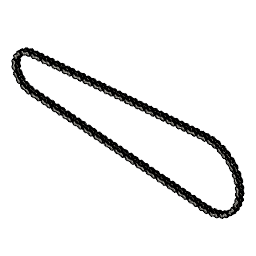
2410994757_Bicycle-Chain (Autodesk Fusion 360 design; units mm, degrees)
part number: 2025-11-01-18-05-41-506
Autodesk Fusion 360 part; units mm, degrees
note: some values were not read from the file. Chosen so that the rebuilt part matches the saved one: a direction; which bodies a step acts on. Set by a fixed rule: which sketch regions a step uses.
sketch "Sketch4" plane through (0, 0, 0) normal (0, 1, 0) x (1, 0, 0)
  line L0 (0, 0) -> (0, -57.0944)
  line L1 (0, 0) -> (-8.7438, -55.2063)
  line L2 (0, 0) -> (8.7438, -55.2063)
  circle A0 centre (0, 0) radius 37.5
  circle A1 centre (-5.8663, -37.0383) radius 4.5
  circle A2 centre (5.8663, -37.0383) radius 4.5
  line L3 (-5.8663, -37.0383) -> (5.8663, -37.0383)
  circle A3 centre (0, -44.8261) radius 5.25
  circle A4 centre (0, -29.2506) radius 5.25
  circle A5 centre (-5.8663, -37.0383) radius 3
  circle A6 centre (-5.8663, -37.0383) radius 2.25
  circle A7 centre (5.8663, -37.0383) radius 2.25
  circle A8 centre (5.8663, -37.0383) radius 3
  dimension "d26" = 9
  dimension "d27" = 9
  dimension "d28" = 75
  dimension "d29" = 9
  dimension "d30" = 10.5
  dimension "d31" = 6
  dimension "d32" = 4.5
  constraint coincident L0.start L1.start
  constraint vertical L0
  constraint coincident A0 A1.centre
  constraint coincident L1 A1.centre
  constraint symmetric L0 A1 A2
  constraint coincident A1.centre L3.start
  constraint coincident A2.centre L3.end
  constraint coincident L0 A3.centre
  constraint tangent A1 A3
  constraint symmetric L3 A3 A4
  constraint concentric A1 A5
  constraint concentric A5 A6
  constraint symmetric L0 A5 A8
  constraint symmetric L0 A6 A7
  measures "d26" angle of L0 L1
  measures "d27" angle of L0 L2
  measures "d28" diameter of A0
  measures "d29" diameter of A1
  measures "d30" diameter of A3
  measures "d31" diameter of A5
  measures "d32" diameter of A6
extrude "Extrude5" add sketch "Sketch4" along normal blind 1.5 contours L0 A2 L3 A4 | L0 A1 L3 A4 | L0 A0 A2 L3 | L0 A0 A1 L3 | L1 A1 L3 A5 | L2 A2 L3 A8 | L1 A0 A1 A5 | L2 A0 A2 A8 | L0 A0 A2 A3 | L0 A0 A1 A3 | A0 A1 L3 A5 | A0 A2 L3 A8 | L1 L3 A5 A6 | L1 A0 A5 A6 | L1 A0 A1 A5 | L2 A0 A7 A8 | L2 L3 A7 A8 | L2 A0 A2 A8 | L1 A0 A1 A5 | L2 A0 A2 A8 | A0 L3 A5 A6 | A0 L3 A7 A8 | L1 A0 A5 A6 | L2 A0 A7 A8 | L1 A0 A5 A6 | L2 A0 A7 A8 makes body 1
extrude "Extrude6" add sketch "Sketch4" along normal mid plane 10.5 separate body contours L1 L3 A6 | L1 A0 A6 | L2 A0 A7 | L2 L3 A7 | A0 L3 A6 | A0 L3 A7 | L1 A0 A6 | L1 A0 A6 | L2 A0 A7 | L2 A0 A7 makes body 2 at (-3.6275, 1.75, 36.8143) makes body 3 at (3.6191, 1.75, 36.9262)
move_body "Align1" bodies 1 to x (1, 0, 0) y (0, 1, 0) z (0, 0, 1) at (0, 3.75, 0)
mirror "Mirror1" about plane through (0, 0, 0) normal (0, 1, 0) of bodies 1 makes body 4
extrude "Extrude7" add sketch "Sketch4" along normal blind 1.5 separate body contours L0 A2 L3 A4 | L0 A1 L3 A4 | L0 A0 A2 L3 | L0 A0 A1 L3 | L1 A1 L3 A5 | L2 A2 L3 A8 | L1 A0 A1 A5 | L2 A0 A2 A8 | L0 A0 A2 A3 | L0 A0 A1 A3 | A0 A1 L3 A5 | A0 A2 L3 A8 | L1 A0 A1 A5 | L2 A0 A2 A8 | L1 A0 A1 A5 | L2 A0 A2 A8 makes body 5
extrude "Extrude8" add sketch "Sketch4" along normal mid plane 7.5 separate body contours L1 L3 A5 A6 | L1 A0 A5 A6 | L2 A0 A7 A8 | L2 L3 A7 A8 | A0 L3 A5 A6 | A0 L3 A7 A8 | L1 A0 A5 A6 | L2 A0 A7 A8 | L1 A0 A5 A6 | L2 A0 A7 A8 makes body 6 at (-2.9075, 2.5, 37.5337) makes body 7 at (8.8514, -1.25, 37.337)
move_body "Align2" bodies 5 to x (1, 0, 0) y (0, 1, 0) z (0, 0, 1) at (0, 2.25, 0)
mirror "Mirror2" about plane through (0, 0, 0) normal (0, 1, 0) of bodies 5 makes body 8
combine "Combine2" operation add target body 5 tool bodies 6 7 8
combine "Combine3" operation add target body 1 tool bodies 2 3 4
move_body "Move1" bodies 1 to x (0.951057, 0, -0.309017) y (0, 1, 0) z (0.309017, 0, 0.951057) at (0, 0, 0)
pattern_circular "C-Pattern2" count 6 over 180 about axis through (0, 0, 0) along (0, -1, 0) of bodies 1 5 makes body 9 at (-17.1688, -5.25, 33.5877) makes body 10 at (-33.5487, -5.25, 17.5808) makes body 11 at (-37.1681, 5.25, 6.1192) makes body 12 at (-27.0874, -5.25, -26.4739) makes body 13 at (-16.7873, -5.25, -33.7221) makes body 14 at (-22.5435, -2.25, 29.403) makes body 15 at (-34.8528, 2.25, 12.5927) makes body 16 at (-34.9303, -2.25, -12.3541) makes body 17 at (-20.9976, -2.25, -30.5262) makes body 18 at (-1.2063, 2.25, -37.0383)
sketch "Sketch5" plane through (0, 0, 0) normal (0, 1, 0) x (1, 0, 0)
  line L0 (0, 0) -> (400, 0)
  line L1 (-3.0469, -37.376) -> (394.3125, -69.7686)
  line L2 (-3.0469, 37.376) -> (394.3125, 69.7686)
  arc A0 (-3.0469, 37.376) -> (-3.0469, -37.376) centre (0, 0) ccw
  arc A1 (394.3125, -69.7686) -> (394.3125, 69.7686) centre (400, 0) ccw
  dimension "d68" = 75
  dimension "d69" = 400
  dimension "d70" = 140
  constraint coincident L0.start A0.centre
  constraint horizontal L0
  constraint coincident L0.end A1.centre
  constraint tangent L1 A0
  constraint tangent L1 A1
  constraint tangent L2 A1
  constraint tangent L2 A0
  measures "d68" diameter of A0
  measures "d69" distance of L0.start L0.end
  measures "d70" diameter of A1
move_body "Move2" bodies 1 to x (1, 0, 0) y (0, 1, 0) z (0, 0, 1) at (100, 0, 0)
move_body "Move3" bodies 5 to x (0.996195, 0, 0.087156) y (0, 1, 0) z (-0.087156, 0, 0.996195) at (2.7965, 0, 1.0273)
move_body "Move4" bodies 5 to x (1, 0, 0) y (0, 1, 0) z (0, 0, 1) at (0.4623, 0, -0.4202)
move_body "Move5" bodies 5 to x (0.999848, 0, 0.017452) y (0, 1, 0) z (-0.017452, 0, 0.999848) at (0.6455, 0, 0.108)
move_body "Move6" bodies 1 to x (1, 0, 0) y (0, 1, 0) z (0, 0, 1) at (-100.03, 0, 1.1325)
move_body "Move7" bodies 1 to x (0.913545, 0, 0.406737) y (0, 1, 0) z (-0.406737, 0, 0.913545) at (16.03, 0, 0.9262)
copy_body "CopyPasteBodies1" bodies 5 makes body 19
move_body "Move8" bodies 19 to x (1, 0, 0) y (0, 1, 0) z (0, 0, 1) at (23.3209, 0, 2.4356)
move_body "Move9" bodies 19 to x (0.999848, 0, -0.017452) y (0, 1, 0) z (0.017452, 0, 0.999848) at (-0.6855, 0, 0.3116)
move_body "Move26" bodies 19 to x (0.999848, 0, -0.017452) y (0, 1, 0) z (0.017452, 0, 0.999848) at (-0.6855, 0, 0.3116)
pattern_path "PathPattern3" count 16 spacing 23.5684 from (17.537, 0, 39.054) backwards path "Sketch5" along L2 A0 L1 A1 of bodies 1 19 makes body 20 at (29.7958, 5.25, 40.9755) makes body 21 at (52.9479, 5.25, 41.8939) makes body 22 at (76.8225, 5.25, 43.3228) makes body 23 at (100.0948, 5.25, 46.0838) makes body 24 at (134.64, 5.25, 49.465) makes body 25 at (146.8849, 5.25, 49.792) makes body 26 at (170.3753, 5.25, 51.7069) makes body 27 at (193.6488, 5.25, 53.9127) makes body 28 at (217.1393, 5.25, 55.8276) makes body 29 at (240.6297, 5.25, 57.7425) makes body 30 at (275.398, -5.25, 59.2453) makes body 31 at (298.8885, -5.25, 61.1603) makes body 32 at (324.347, 5.25, 65.2814) makes body 33 at (345.9825, 5.25, 65.0292) makes body 34 at (370.9655, 5.25, 70.5162) makes body 35 at (48.3035, 3.75, 41.8554) makes body 36 at (71.794, 3.75, 43.7704) makes body 37 at (95.2845, 3.75, 45.6853) makes body 38 at (118.775, 3.75, 47.6002) makes body 39 at (142.2655, 3.75, 49.5152) makes body 40 at (165.756, 3.75, 51.4301) makes body 41 at (189.2465, 3.75, 53.345) makes body 42 at (212.737, 3.75, 55.26) makes body 43 at (236.2275, 3.75, 57.1749) makes body 44 at (259.718, 3.75, 59.0898) makes body 45 at (283.2085, 3.75, 61.0048) makes body 46 at (306.6989, 3.75, 62.9197) makes body 47 at (330.1894, 3.75, 64.8346) makes body 48 at (353.6799, 3.75, 66.7496) makes body 49 at (377.1704, 3.75, 68.6645)
copy_body "CopyPasteBodies8" bodies 49 makes body 50
move_body "Move27" bodies 50 to x (1, 0, 0) y (0, 1, 0) z (0, 0, 1) at (0.2451, 0, 16.7885)
copy_body "CopyPasteBodies9" bodies 34 makes body 51
move_body "Move28" bodies 51 to x (1, 0, 0) y (0, 1, 0) z (0, 0, 1) at (23.3972, 0, 2.0954)
move_body "Move29" bodies 51 to x (0.99863, 0, -0.052336) y (0, 1, 0) z (0.052336, 0, 0.99863) at (-3.0868, 0, 20.0643)
move_body "Move30" bodies 50 to x (1, 0, 0) y (0, 1, 0) z (0, 0, 1) at (23.1694, 0, -15.3208)
move_body "Move31" bodies 50 to x (0.99863, 0, -0.052336) y (0, 1, 0) z (0.052336, 0, 0.99863) at (-3.1047, 0, 20.6781)
copy_body "CopyPasteBodies10" bodies 51 makes body 52
move_body "Move32" bodies 52 to x (1, 0, 0) y (0, 1, 0) z (0, 0, 1) at (23.4006, 0, 0.8481)
move_body "Move33" bodies 52 to x (0.978148, 0, -0.207912) y (0, 1, 0) z (0.207912, 0, 0.978148) at (-5.6699, 0, 85.7287)
pattern_circular "C-Pattern4" count 10 over 178 about axis through (400, 0, 0) along (0, 1, 0) of bodies 50 52 makes body 53 at (421.884, -2.25, 66.2075) makes body 54 at (444.6864, 2.25, 53.5498) makes body 55 at (460.0112, -3.75, 35.4663) makes body 56 at (468.4721, -3.75, 13.0681) makes body 57 at (468.8528, 2.25, -11.1243) makes body 58 at (461.1146, -3.75, -33.5292) makes body 59 at (447.5941, -2.25, -50.9622) makes body 60 at (425.7675, -3.75, -64.7706) makes body 61 at (402.3309, -3.75, -69.669) makes body 62 at (439.7015, -5.25, 58.838) makes body 63 at (457.1988, -5.25, 41.6673) makes body 64 at (461.6259, -5.25, 31.2474) makes body 65 at (469.8678, 5.25, 8.1663) makes body 66 at (464.7607, 5.25, -26.7914) makes body 67 at (458.9149, -5.25, -37.8234) makes body 68 at (442.0521, -5.25, -54.3687) makes body 69 at (421.0095, -5.25, -66.9915) makes body 70 at (397.3154, 5.25, -70.0733)
move_body "Move34" bodies 18 to x (0.996195, 0, -0.087156) y (0, 1, 0) z (0.087156, 0, 0.996195) at (3.2058, 0, -0.6522)
copy_body "CopyPasteBodies11" bodies 13 makes body 71
move_body "Move35" bodies 71 to x (1, 0, 0) y (0, 1, 0) z (0, 0, 1) at (22.8302, 0, -4.6624)
move_body "Move36" bodies 71 to x (0.97437, 0, 0.224951) y (0, 1, 0) z (-0.224951, 0, 0.97437) at (-8.4126, 0, -2.2851)
copy_body "CopyPasteBodies12" bodies 18 makes body 72
move_body "Move37" bodies 72 to x (1, 0, 0) y (0, 1, 0) z (0, 0, 1) at (23.3544, 0, -2.0564)
pattern_path "PathPattern4" count 16 spacing 23.8027 from (17.4965, 0, -39.0507) backwards path "Sketch5" along A1 L1 A0 L2 of bodies 71 72 makes body 73 at (40.8818, 5.25, -41.2269) makes body 74 at (53.4216, 5.25, -41.6188) makes body 75 at (77.2852, 5.25, -43.9069) makes body 76 at (101.0092, 5.25, -45.8409) makes body 77 at (135.8164, 5.25, -48.5228) makes body 78 at (159.7125, -5.25, -50.8138) makes body 79 at (172.0417, -5.25, -51.2886) makes body 80 at (195.7658, -5.25, -53.2226) makes body 81 at (230.8846, -5.25, -56.6157) makes body 82 at (254.4366, -5.25, -58.1927) makes body 83 at (277.8561, -5.25, -59.3077) makes body 84 at (289.6933, -5.25, -61.7724) makes body 85 at (313.4174, -5.25, -63.7064) makes body 86 at (336.0601, -5.25, -65.7366) makes body 87 at (362.2998, -5.25, -66.3041) makes body 88 at (45.8544, 2.25, -41.4348) makes body 89 at (69.5784, 2.25, -43.3688) makes body 90 at (93.5547, -3.75, -45.2922) makes body 91 at (117.2787, -3.75, -47.2262) makes body 92 at (140.7505, 2.25, -49.1707) makes body 93 at (164.4746, 2.25, -51.1047) makes body 94 at (188.1986, 2.25, -53.0387) makes body 95 at (211.9226, 2.25, -54.9726) makes body 96 at (235.6466, 2.25, -56.9066) makes body 97 at (259.3707, 2.25, -58.8406) makes body 98 at (285.2482, -2.25, -60.9629) makes body 99 at (308.9722, -2.25, -62.8969) makes body 100 at (332.6962, -2.25, -64.8309) makes body 101 at (356.4203, -2.25, -66.7649) makes body 102 at (380.1443, -2.25, -68.6988)
move_body "Move38" bodies 70 to x (0.996195, 0, 0.087156) y (0, 1, 0) z (-0.087156, 0, 0.996195) at (-4.5858, 0, -34.9061)
equation "d35 = ( 3.5 * 1.5 ) * 1 mm"
equation "d41 = ( 2.5 * 1.5 ) * 1 mm"
